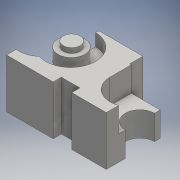
# Autodesk Inventor part: 240626_part1
Saved by Autodesk Inventor 2016 (Build 200138000, 138)
## iProperties
Created: 2024-06-26
Part Number: 240626_part1
Material: 일반
Document SubType Name: Modeling
Designer: pc
Density: 1 g/cm^3
Appearance: 기본값
Author: pc
Autodesk Inventor part; units mm, degrees
ref_plane "YZ Plane" through (0, 0, 0) normal (1, 0, 0) x (0, 1, 0)
ref_plane "XZ Plane" through (0, 0, 0) normal (0, 1, 0) x (-1, 0, 0)
ref_plane "XY Plane" through (0, 0, 0) normal (0, 0, 1) x (1, 0, 0)
sketch "스케치1" plane through (0, 0, 0) normal (0, 0, 1) x (1, 0, 0)
  line L0 (20.2592, -13.6377) -> (-20.2592, -13.6377)
  line L1 (-20.2592, -13.6377) -> (-20.2592, 13.6377)
  line L2 (-20.2592, 13.6377) -> (20.2592, 13.6377)
  line L3 (20.2592, 13.6377) -> (20.2592, -13.6377)
  line L4 (20.2592, -13.6377) -> (-20.2592, 13.6377) construction
  line L5 (-20.2592, -13.6377) -> (20.2592, 13.6377) construction
  point P0 (0, 0)
  constraints: 12 end point, 2 midpoint, 2 parallel, 1 horizontal, 1 perpendicular
extrude "돌출1" add sketch "스케치1" along normal blind 20
sketch "스케치2" plane through (0, 0, 20) normal (0, 0, 1) x (1, 0, 0)
  line L0 (20.2592, 13.6377) -> (-20.2592, 13.6377) projected
  line L1 (-10.0264, 13.6377) -> (-10.0264, -1.4111)
  line L2 (-20.2592, 13.6377) -> (-20.2592, -13.6377) projected
  arc A0 (-20.2592, -9.7293) -> (-10.0264, -1.4111) centre (-19.2526, -0.5144) ccw
  line L3 (-10.0264, 13.6377) -> (-20.2592, 13.6377)
  line L4 (-20.2592, -9.7293) -> (-20.2592, 13.6377)
  line L5 (7.8725, 13.6377) -> (20.2592, 13.6377)
  line L6 (20.2592, 13.6377) -> (20.2592, 8.2439)
  line L7 (20.2592, 8.2439) -> (7.8725, 8.2439)
  line L8 (7.8725, 8.2439) -> (7.8725, 13.6377)
  point P0 (0, 0)
  constraints: 14 end point, 3 perpendicular, 3 point on line, 2 parallel, 2 point on circle, 1 centre point, 1 collinear, 1 horizontal
extrude "돌출2" cut sketch "스케치2" against normal blind 20
sketch "스케치3" plane through (0, 0, 20) normal (0, 0, 1) x (1, 0, 0)
  line L0 (-10.0264, -1.4111) -> (-10.0264, 13.6377) projected
  circle A0 centre (-10.0264, 2.161) radius 10.136
  line L1 (20.2592, 8.2439) -> (20.2592, -13.6377) projected
  line L2 (20.2592, 7.0816) -> (20.2592, -8.6286)
  line L3 (8.5169, 7.0816) -> (8.5169, -0.7735)
  arc A1 (8.5169, -0.7735) -> (20.2592, -8.6286) centre (17.3236, -0.3127) ccw
  line L4 (8.5169, 7.0816) -> (8.5169, 8.2439)
  line L5 (8.5169, 8.2439) -> (20.2592, 8.2439)
  point P0 (0, 0)
  constraints: 8 end point, 3 point on line, 2 centre point, 2 point on circle, 2 vertical, 1 perpendicular
extrude "돌출3" cut sketch "스케치3" against normal blind 5 contours A0
extrude "돌출4" cut sketch "스케치3" against normal blind 10 contours L1 A1 L3 L4 L5
sketch "스케치4" plane through (0, 0, 15) normal (0, 0, 1) x (1, 0, 0)
  line L0 (-10.0264, -1.4111) -> (-10.0264, 12.2971) projected
  circle A0 centre (-10.0264, 2.488) radius 5.4337
  point P0 (0, 0)
  constraints: 1 centre point, 1 point on line
extrude "돌출5" add sketch "스케치4" along normal blind 5
sketch "스케치5" plane through (-10.0264, 2.488, 20) normal (0, 0, 1) x (1, 0, 0)
  line L0 (0, -3.8991) -> (0, 5.4337) projected
  circle A0 centre (0, 0.0967) radius 3.434
  point P0 (10.0264, -2.488)
  constraints: 1 centre point, 1 point on line
extrude "돌출6" add sketch "스케치5" along normal blind 2
sketch "스케치6" plane through (0, 0, 10) normal (0, 0, 1) x (1, 0, 0)
  line L0 (20.2592, 8.2439) -> (20.2592, -13.6377) projected
  circle A0 centre (20.2592, 0) radius 5.9354
  point P0 (0, 0)
  constraints: 1 centre point, 1 point on line
extrude "돌출7" cut sketch "스케치6" against normal blind 20
sketch "스케치7" plane through (0, 0, 20) normal (0, 0, 1) x (1, 0, 0)
  line L0 (20.2592, -13.6377) -> (-20.2592, -13.6377) projected
  line L1 (-1.3274, -10.3147) -> (6.1983, -10.3147)
  line L2 (6.1983, -10.3147) -> (6.1983, -13.6377)
  line L3 (6.1983, -13.6377) -> (-1.3274, -13.6377)
  line L4 (-1.3274, -13.6377) -> (-1.3274, -10.3147)
  point P0 (0, 0)
  constraints: 8 end point, 2 parallel, 1 horizontal, 1 perpendicular, 1 point on line
extrude "돌출8" cut sketch "스케치7" against normal blind 20
